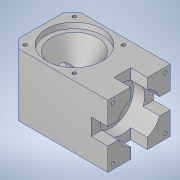
# Autodesk Inventor part: MC18_KörperEigen
Saved by Autodesk Inventor 2021 (Build 250183000, 183)
## iProperties
Created: 2020-04-27
Part Number: MC18_KörperEigen
Material: Aluminium 6061
Document SubType Name: Modeling
Designer: kaebi
Density: 2.7 g/cm^3
Appearance: Aluminium - flach
Description: Körper
Stock Number: BEF 011 A
Mass: 527.347 g
Surface Area: 331.56 cm^2
Volume: 195.314 cm^3
Author: kaebi
Autodesk Inventor part; units mm, degrees
note: some values were not read from the file. Chosen so that the rebuilt part matches the saved one: direction of "Bohrung3".
ref_plane "YZ Plane" through (0, 0, 0) normal (1, 0, 0) x (0, 1, 0)
ref_plane "XZ Plane" through (0, 0, 0) normal (0, 1, 0) x (-1, 0, 0)
ref_plane "XY Plane" through (0, 0, 0) normal (0, 0, 1) x (1, 0, 0)
sketch "Skizze1" plane through (0, 0, 0) normal (0, 0, 1) x (1, 0, 0)
  line L0 (0, 28) -> (88, 28)
  line L1 (88, 28) -> (88, -28)
  line L2 (88, -28) -> (42, -28)
  line L3 (42, -28) -> (30, -15)
  line L4 (30, -15) -> (0, -15)
  line L5 (0, -15) -> (0, 28)
  point P0 (0, 0)
  point P1 (88, 0)
  dimension "d0" = 88
  dimension "d1" = 43
  dimension "d2" = 56
  dimension "d3" = 30
  dimension "d4" = 12
  constraints: 12 end point, 3 perpendicular, 1 horizontal, 1 horizontal alignment, 1 midpoint, 1 parallel, 1 vertical alignment
  measures "d0" distance of L0.start L0.end
  measures "d1" distance of L4.end L0.start
  measures "d2" distance of L0.end L1.end
  measures "d3" distance of L3.end L4.end
  measures "d4" horizontal distance of L2.end L3.end
extrude "Extrusion1" add sketch "Skizze1" along normal mid plane 56
sketch "Skizze3" plane through (0, 0, 0) normal (0, 0, 1) x (1, 0, 0)
  line L0 (88, 28) -> (0, 28) projected
  line L1 (5, 28) -> (5, 23)
  line L2 (5, 23) -> (9, 23)
  line L3 (9, 23) -> (22.5, 0)
  line L4 (22.5, 0) -> (30, 0)
  line L5 (30, 0) -> (30, 28)
  line L6 (5, 28) -> (30, 28)
  line L7 (30, 43.7054) -> (30, 36.9492)
  line L8 (0, -15) -> (0, 28) projected
  line L9 (88, 28) -> (88, -28) projected
  point P0 (0, 0)
  point P1 (88, 0)
  point P2 (0, -28)
  dimension "d7" = 30
  dimension "d8" = 50
  dimension "d9" = 4
  dimension "d10" = 15
  dimension "d11" = 5
  constraints: 14 end point, 3 perpendicular, 2 point on line, 2 vertical, 1 collinear, 1 horizontal alignment, 1 midpoint, 1 parallel
  measures "d7" distance between parallel lines of L8 L7
  measures "d8" diameter of L1 L7
  measures "d9" distance of L1.end L2.end
  measures "d10" diameter of L3.end L7
  measures "d11" distance of L1.start L1.end
revolve "Umdrehung1" cut sketch "Skizze3" angle 360 about axis through (30, 43.7054, 0) along (0, -1, 0)
sketch "Skizze4" plane through (0, 28, 28) normal (0, 1, 0) x (1, 0, 0)
  line L0 (8, 6) -> (52, 6)
  line L1 (52, 6) -> (52, 50)
  line L2 (52, 50) -> (8, 50)
  line L3 (8, 50) -> (8, 6)
  line L4 (8, 6) -> (52, 50) construction
  line L5 (52, 6) -> (8, 50) construction
  circle A0 centre (30, 28) radius 25 projected
  point P0 (0, 28)
  point P1 (30, 28)
  point P2 (30, 28)
  dimension "d13" = 44
  constraints: 12 end point, 5 coincident, 3 midpoint, 2 parallel, 2 perpendicular, 1 horizontal
  measures "d13" distance of L1.end L2.end
hole "Bohrung1" at (8, 28, -22) at (52, 28, -22) at (52, 28, 22) at (8, 28, 22) direction (0, -1, 0) diameter 3.242 depth 13 tip angle 118 thread size "M4x0.7" class "6H" standard "ISO Metric profile"
sketch "Skizze6" plane through (88, -28, 28) normal (1, 0, 0) x (0, 0, -1)
  circle A0 centre (28, 28) radius 7.75
  dimension "d24" = 15.5
  constraints: 1 centre point, 1 coincident
  measures "d24" diameter of A0
extrude "Extrusion3" cut sketch "Skizze6" against normal through all
sketch "Skizze7" plane through (0, -15, 28) normal (-1, 0, 0) x (0, 0, 1)
  circle A0 centre (-28, 15) radius 9
  circle A1 centre (-28, 15) radius 7.75 projected
  dimension "d27" = 18
  constraints: 1 centre point, 1 concentric
  measures "d27" diameter of A0
extrude "Extrusion4" cut sketch "Skizze7" against normal blind 15
sketch "Skizze8" plane through (88, -28, 28) normal (1, 0, 0) x (0, 0, -1)
  circle A0 centre (28, 28) radius 20
  dimension "d30" = 40
  constraints: 1 centre point, 1 coincident
  measures "d30" diameter of A0
extrude "Extrusion5" cut sketch "Skizze8" against normal blind 25
sketch "Skizze9" plane through (88, -28, 28) normal (1, 0, 0) x (0, 0, -1)
  line L0 (4.45, 4.45) -> (51.55, 4.45)
  line L1 (51.55, 4.45) -> (51.55, 51.55)
  line L2 (51.55, 51.55) -> (4.45, 51.55)
  line L3 (4.45, 51.55) -> (4.45, 4.45)
  circle A0 centre (28, 28) radius 9 projected
  line L4 (4.45, 4.45) -> (51.55, 51.55) construction
  line L5 (51.55, 4.45) -> (4.45, 51.55) construction
  dimension "d33" = 47.1
  dimension "d34" = 47.1
  constraints: 12 end point, 4 coincident, 2 midpoint, 2 parallel, 1 horizontal, 1 perpendicular
  measures "d33" distance of L1.end L2.end
  measures "d34" distance between parallel lines of L0 L2
hole "Bohrung2" at (88, 23.55, 23.55) at (88, -23.55, -23.55) at (88, -23.55, 23.55) at (88, 23.55, -23.55) direction (-1, 0, 0) diameter 3.242 depth 13 tip angle 118 thread size "M4x0.7" class "6H" standard "ISO Metric profile"
sketch "Skizze10" plane through (88, -28, 28) normal (1, 0, 0) x (0, 0, -1)
  line L0 (0, 20.5) -> (56, 20.5)
  line L1 (56, 20.5) -> (56, 35.5)
  line L2 (56, 35.5) -> (0, 35.5)
  line L3 (0, 35.5) -> (0, 20.5)
  line L4 (0, 20.5) -> (56, 35.5) construction
  line L5 (56, 20.5) -> (0, 35.5) construction
  line L6 (20.5, 0) -> (35.5, 0)
  line L7 (35.5, 0) -> (35.5, 56)
  line L8 (35.5, 56) -> (20.5, 56)
  line L9 (20.5, 56) -> (20.5, 0)
  line L10 (20.5, 0) -> (35.5, 56) construction
  line L11 (35.5, 0) -> (20.5, 56) construction
  line L12 (0, 56) -> (56, 56) projected
  line L13 (56, 56) -> (56, 0) projected
  point P0 (28, 28)
  dimension "d42" = 15
  constraints: 24 end point, 4 midpoint, 4 parallel, 3 perpendicular, 2 collinear, 2 horizontal
  measures "d42" distance of L7.end L8.end
extrude "Extrusion6" cut sketch "Skizze10" against normal blind 15 contours L3 L2 L9 L0 | L9 L2 L7 L0 | L0 L7 L6 L9 | L7 L2 L1 L0 | L9 L8 L7 L2
sketch "Skizze12" plane through (0, 0, 28) normal (0, 0, 1) x (1, 0, 0)
  line L0 (0, -15) -> (30, -15) projected
  line L1 (30, -15) -> (42, -28) projected
  line L2 (42, -28) -> (88, -28) projected
  line L3 (88, -28) -> (88, -7.5) projected
  line L4 (88, -7.5) -> (73, -7.5) projected
  line L5 (73, -7.5) -> (73, 7.5) projected
  line L6 (73, 7.5) -> (88, 7.5) projected
  line L7 (88, 7.5) -> (88, 28) projected
  line L8 (88, 28) -> (0, 28) projected
  line L9 (0, -15) -> (8, -15) projected
  line L10 (8, -15) -> (8, 28) projected
  line L11 (8, 28) -> (0, 28) projected
  line L12 (0, 28) -> (0, -15) projected
  line L13 (42, -28) -> (30, -15)
  line L14 (0, -15) -> (0, -28)
  line L15 (0, -28) -> (42, -28)
  line L16 (30, -15) -> (0, -15)
  line L17 (0, 28) -> (0, -15) projected
  constraints: 8 end point, 2 collinear, 1 perpendicular, 1 vertical
extrude "Extrusion7" add sketch "Skizze12" against normal up to surface (56 mm away) contours L0 L1 L15 L14
sketch "Skizze11" plane through (0, -28, 28) normal (0, -1, 0) x (1, 0, 0)
  line L0 (73, -20.5) -> (88, -20.5) projected
  line L1 (88, 0) -> (88, -20.5) projected
  line L2 (0, 0) -> (88, 0) projected
  line L3 (0, 0) -> (0, -56) projected
  line L4 (88, -56) -> (0, -56) projected
  line L5 (88, -35.5) -> (88, -56) projected
  line L6 (88, -35.5) -> (73, -35.5) projected
  line L7 (73, -35.5) -> (73, -20.5) projected
  point P0 (0, -28)
  point P1 (5, -28)
  point P2 (0, -28)
  point P3 (73, -28)
  dimension "d61" = 5
  constraints: 2 horizontal alignment, 1 midpoint
  measures "d61" distance from line of L3 point (5, -28)
hole "Bohrung3" at (5, -28, 0) direction (0, 1, 0) diameter 3.242 end up to surface thread size "M4x0.7" class "6H" standard "ISO Metric profile"
chamfer "Fase2" distance 8 angle 45 2 edges at (0, 0, -28) (0, 0, 28)
